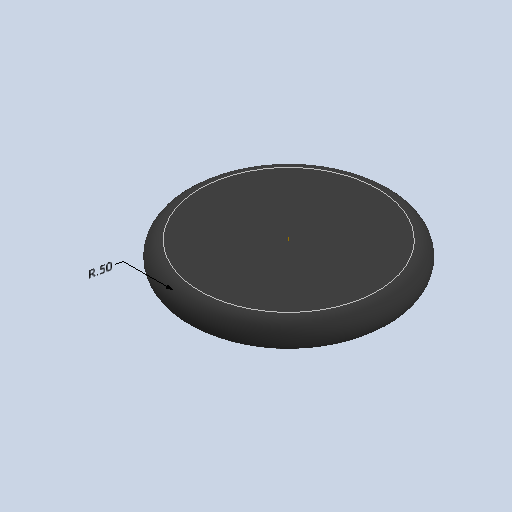
# Autodesk Inventor part: RS-01
Saved by Autodesk Inventor 2022 (Build 260153000, 153)
## iProperties
Company: El Camino College
Created: 2023-05-15
Part Number: RS-01
Material: Rubber, Silicone
Document SubType Name: Modeling
Designer: Edgar Tejada
Density: 1.25 g/cm^3
Appearance: Rubber - Black
Project: Hexagonal Hive
Mass: 797.105 g
Surface Area: 615.117 cm^2
Volume: 637.684 cm^3
Description: Silicone Stopper for Insulation and Sealing Lid
Author: Edgar Tejada
Title: Rubber Stoper
Subject: Hexagonal Hive
Autodesk Inventor part; units mm, degrees
ref_plane "YZ Plane" through (0, 0, 0) normal (1, 0, 0) x (0, 1, 0)
ref_plane "XZ Plane" through (0, 0, 0) normal (0, 1, 0) x (-1, 0, 0)
ref_plane "XY Plane" through (0, 0, 0) normal (0, 0, 1) x (1, 0, 0)
sketch "Sketch1" plane through (0, 0, 0) normal (0, 1, 0) x (-1, 0, 0)
  circle A0 centre (0, 0) radius 92.075
  dimension "d0" = 184.15
  constraints: 1 centre point, 1 coincident
  measures "d0" diameter of A0
extrude "Extrusion1" add sketch "Sketch1" along normal blind 25.4
fillet "Fillet1" radius 12.7 2 edges at (92.075, 25.4, 0) (92.075, 0, 0)
body "Solid1"
